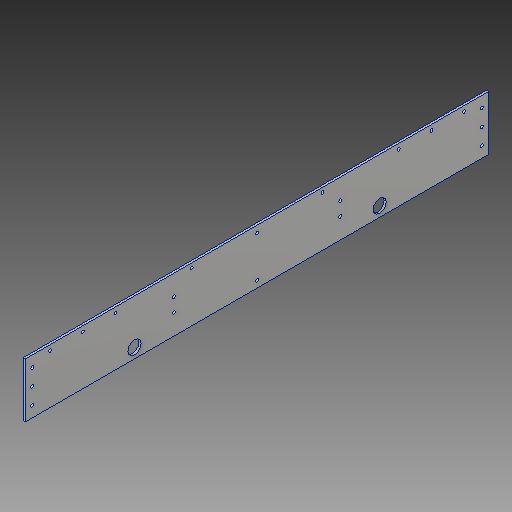
# Autodesk Inventor part: Bumper Plate
Saved by Autodesk Inventor 2019.4 (Build 234330000, 330)
## iProperties
Created: 2019-11-03
Part Number: Bumper Plate
Material: Aluminum 6061
Document SubType Name: Modeling
Designer: admin
Density: 2.7 g/cm^3
Appearance: Aluminum - Flat
Mass: 902.933 g
Surface Area: 1768 cm^2
Volume: 334.42 cm^3
Author: admin
Autodesk Inventor part; units mm, degrees
ref_plane "YZ Plane" through (0, 0, 0) normal (1, 0, 0) x (0, 1, 0)
ref_plane "XZ Plane" through (0, 0, 0) normal (0, 1, 0) x (-1, 0, 0)
ref_plane "XY Plane" through (0, 0, 0) normal (0, 0, 1) x (1, 0, 0)
sketch "Sketch1" plane through (0, 0, 0) normal (1, 0, 0) x (0, 1, 0)
  line L0 (-50, 425) -> (50, 425)
  line L1 (50, 425) -> (50, -425)
  line L2 (50, -425) -> (-50, -425)
  line L3 (-50, -425) -> (-50, 425)
  line L4 (-50, 425) -> (50, -425) construction
  line L5 (50, 425) -> (-50, -425) construction
  point P0 (0, 0)
  dimension "d0" = 100
  dimension "d1" = 850
  constraints: 12 end point, 2 midpoint, 2 parallel, 1 horizontal, 1 perpendicular
  measures "d0" distance of L1.end L2.end
  measures "d1" distance of L0.end L1.end
extrude "Extrusion1" add sketch "Sketch1" along normal blind 4
sketch "Sketch2" plane through (4, 0, 0) normal (1, 0, 0) x (0, 0, -1)
  circle A0 centre (-225, -31.7) radius 12.1
  line L0 (-425, -50) -> (425, -50) projected
  line L1 (-425, 50) -> (-425, -50) projected
  line L2 (425, 50) -> (-425, 50) projected
  line L3 (0, 50) -> (0, -50)
  circle A1 centre (225, -31.7) radius 12.1
  point P0 (0, 0)
  dimension "d4" = 18.3
  dimension "d5" = 200
  dimension "d6" = 24.2
  dimension "d9" = 425
  constraints: 2 centre point, 2 end point, 2 midpoint, 1 perpendicular, 1 symmetric about line, 1 other
  measures "d4" distance from line of L0 A0.centre
  measures "d5" distance from line of L1 A0.centre
  measures "d6" diameter of A0
  measures "d9" distance between parallel lines of L1 L3
extrude "Extrusion2" cut sketch "Sketch2" against normal through all contours A0 | A1
sketch "Sketch3" plane through (4, 0, 0) normal (1, 0, 0) x (0, 0, -1)
  circle A0 centre (120, -42) radius 2.75 projected
  circle A1 centre (120, 42) radius 2.75 projected
  circle A2 centre (0, 37.5) radius 2.75 projected
  circle A3 centre (412.5, 30) radius 2.75 projected
  circle A4 centre (412.5, 0) radius 2.75 projected
  circle A5 centre (412.5, -30) radius 2.75 projected
  circle A6 centre (260, 40.5) radius 2.75 projected
  circle A7 centre (320, 40.5) radius 2.75 projected
  circle A8 centre (145.213, 6.296) radius 10.5 projected
  circle A9 centre (196.913, 6.296) radius 10.5 projected
  circle A10 centre (-145.213, 6.296) radius 10.5 projected
  circle A11 centre (-196.913, 6.296) radius 10.5 projected
  circle A12 centre (-105, -14) radius 10 projected
  circle A13 centre (-79.6, -14) radius 2.75 projected
  circle A14 centre (-130.4, -14) radius 2.75 projected
  circle A15 centre (-264.9997, -22.6996) radius 2.75 projected
  circle A16 centre (-147.163, -33.4172) radius 2.75 projected
  circle A17 centre (264.9997, -22.6996) radius 2.75 projected
  circle A18 centre (174.913, 42.776) radius 2.75 projected
  circle A19 centre (147.163, -33.4172) radius 2.75 projected
  circle A20 centre (130.4, -14) radius 2.75 projected
  circle A21 centre (79.6, -14) radius 2.75 projected
  circle A22 centre (105, 11.4) radius 2.75 projected
  circle A23 centre (105, -39.4) radius 2.75 projected
  circle A24 centre (111.5777, 29.8129) radius 2.75 projected
  circle A25 centre (236.913, 19.219) radius 2.75 projected
  circle A26 centre (-236.913, 19.219) radius 2.75 projected
  circle A27 centre (-174.913, 42.776) radius 2.75 projected
  circle A28 centre (-111.5777, 29.8129) radius 2.75 projected
  circle A29 centre (-105, 11.4) radius 2.75 projected
  circle A30 centre (-105, -39.4) radius 2.75 projected
  circle A31 centre (241, -31.7) radius 2.25 projected
  circle A32 centre (-241, -31.7) radius 2.25 projected
  circle A33 centre (-209, -31.7) radius 2.25 projected
  circle A34 centre (-225, -15.7) radius 2.25 projected
  circle A35 centre (225, -15.7) radius 2.25 projected
  circle A36 centre (209, -31.7) radius 2.25 projected
  circle A37 centre (-225, -31.7) radius 12.3 projected
  circle A38 centre (225, -31.7) radius 12.3 projected
  line L0 (-425, 50) -> (-425, -50) projected
  line L1 (-425, 50) -> (425, 50) projected
  line L2 (425, -50) -> (425, 50) projected
  line L3 (-425, -50) -> (425, -50) projected
  circle A39 centre (-152.5, 12.5) radius 2.75 projected
  circle A40 centre (152.5, 12.5) radius 2.75 projected
  circle A41 centre (152.5, -12.5) radius 2.75 projected
  circle A42 centre (-152.5, -12.5) radius 2.75 projected
  circle A43 centre (0, -37.5) radius 2.75 projected
  circle A44 centre (320, 40.5) radius 2.75 projected
  circle A45 centre (260, 40.5) radius 2.75 projected
  circle A46 centre (0, 37.5) radius 2.75 projected
  circle A47 centre (120, 42) radius 2.75 projected
  circle A48 centre (380, 40.5) radius 2.75 projected
  circle A49 centre (412.5, 0) radius 2.75 projected
  circle A50 centre (412.5, -30) radius 2.75 projected
  circle A51 centre (-264.9997, -22.6996) radius 2.75 projected
  circle A52 centre (-147.163, -33.4172) radius 2.75 projected
  circle A53 centre (264.9997, -22.6996) radius 2.75 projected
  circle A54 centre (174.913, 42.776) radius 2.75 projected
  circle A55 centre (147.163, -33.4172) radius 2.75 projected
  circle A56 centre (111.5777, 29.8129) radius 2.75 projected
  circle A57 centre (236.913, 19.219) radius 2.75 projected
  circle A58 centre (-236.913, 19.219) radius 2.75 projected
  circle A59 centre (-174.913, 42.776) radius 2.75 projected
  circle A60 centre (-111.5777, 29.8129) radius 2.75 projected
  circle A61 centre (225, -31.7) radius 16.3 projected
  circle A62 centre (-225, -31.7) radius 16.3 projected
  line L4 (-425, -50) -> (-425, 50) projected
  line L5 (-425, -50) -> (425, -50) projected
  line L6 (425, 50) -> (425, -50) projected
  line L7 (-425, 50) -> (425, 50) projected
  circle A63 centre (-120, 42) radius 2.75 projected
  circle A64 centre (-105, -14) radius 34 projected
  circle A65 centre (75.0667, -42) radius 2.75 projected
  circle A66 centre (105, -14) radius 34 projected
  circle A67 centre (152.5, -12.5) radius 7.5 projected
  circle A68 centre (-152.5, -12.5) radius 7.5 projected
  circle A69 centre (-85.6, 40) radius 2.75 projected
  circle A70 centre (15.6, 40) radius 2.75 projected
  circle A71 centre (364.4, 40) radius 2.75 projected
  circle A72 centre (364.5, -40) radius 2.75 projected
  circle A73 centre (15.6, -40) radius 2.75 projected
  circle A74 centre (-85.6, -40) radius 2.75 projected
  arc A75 (-119.576, -44.7171) -> (-92.3554, -45.5613) centre (-105, -14) ccw projected
  circle A76 centre (15.6, -40) radius 8.75 projected
  circle A77 centre (-85.6, 40) radius 8.75 projected
  circle A78 centre (15.6, 40) radius 8.75 projected
  circle A79 centre (364.5, -40) radius 8.75 projected
  arc A80 (-92.3554, -45.5613) -> (-78.3455, -35.1077) centre (-85.6, -40) ccw projected
  circle A81 centre (105, -14) radius 10 projected
  circle A82 centre (0, 0) radius 25 projected
  circle A83 centre (0, 0) radius 25 projected
  arc A84 (119.576, -44.7171) -> (122.4969, -43.1523) centre (120, -42) ccw projected
  arc A85 (122.4969, -43.1523) -> (119.576, -44.7171) centre (105, -14) ccw projected
  arc A86 (-78.3455, -35.1077) -> (-122.4969, -43.1523) centre (-105, -14) ccw projected
  circle A87 centre (412.5, 30) radius 2.75 projected
  circle A88 centre (412.5, 30) radius 2.75 projected
  circle A89 centre (364.4, 40) radius 8.75 projected
  circle A90 centre (364.4, 40) radius 8.75 projected
  circle A91 centre (0, -37.5) radius 7.75 projected
  circle A92 centre (380, 40.5) radius 6.75 projected
  circle A93 centre (-412.5, 0) radius 2.75 projected
  circle A94 centre (-380, 40.5) radius 2.75 projected
  circle A95 centre (-260, 40.5) radius 2.75 projected
  circle A96 centre (-320, 40.5) radius 2.75 projected
  circle A97 centre (-412.5, 30) radius 2.75 projected
  circle A98 centre (-412.5, -30) radius 2.75 projected
  circle A99 centre (-120, -42) radius 2.75 projected
  arc A100 (-122.4969, -43.1523) -> (-119.576, -44.7171) centre (-120, -42) ccw projected
  circle A101 centre (-412.5, -30) radius 2.75 projected
  circle A102 centre (-412.5, 30) radius 2.75 projected
  circle A103 centre (-320, 40.5) radius 2.75 projected
  circle A104 centre (-260, 40.5) radius 2.75 projected
  circle A105 centre (-380, 40.5) radius 2.75 projected
  circle A106 centre (-412.5, 0) radius 2.75 projected
  circle A107 centre (-120, 42) radius 2.75 projected
  point P0 (0, 0)
  point P1 (72.4969, -43.1523)
  point P2 (69.576, -44.7171)
  point P3 (369.0669, 32.5985)
  point P4 (365.7758, 31.3588)
  point P5 (368.1667, 30)
  point P6 (-105, -14)
  point P7 (-105, -14)
  point P8 (105, -14)
  point P9 (-105, -14)
  point P10 (-105, -14)
  constraints: 2 other
extrude "Extrusion3" cut sketch "Sketch3" against normal blind 10 contours A1 | A2 | A4 | A5 | A6 | A7 | A40 A8 | A8 A40 | A39 A10 | A10 A39 | A41 | A42 | A43 picked at (152.3295, 12.2121) picked at (153.6603, 13.4669) picked at (-152.2792, 12.2624) picked at (-153.718, 13.3887)
sketch "Sketch4" plane through (4, 0, 0) normal (1, 0, 0) x (0, 0, -1)
  circle A0 centre (120, 42) radius 2.75 projected
  circle A1 centre (0, 37.5) radius 2.75 projected
  circle A2 centre (-120, 42) radius 2.75 projected
  circle A3 centre (152.5, 12.5) radius 2.75 projected
  circle A4 centre (152.5, -12.5) radius 2.75 projected
  circle A5 centre (-152.5, 12.5) radius 2.75 projected
  circle A6 centre (-152.5, -12.5) radius 2.75 projected
  circle A7 centre (-412.5, 30) radius 2.75 projected
  circle A8 centre (-412.5, 0) radius 2.75 projected
  circle A9 centre (-412.5, -30) radius 2.75 projected
  circle A10 centre (412.5, 30) radius 2.75 projected
  circle A11 centre (412.5, 0) radius 2.75 projected
  circle A12 centre (412.5, -30) radius 2.75 projected
  circle A13 centre (380, 40.5) radius 2.75 projected
  circle A14 centre (320, 40.5) radius 2.75 projected
  circle A15 centre (260, 40.5) radius 2.75 projected
  circle A16 centre (-380, 40.5) radius 2.75 projected
  circle A17 centre (-320, 40.5) radius 2.75 projected
  circle A18 centre (-260, 40.5) radius 2.75 projected
  point P0 (0, 0)
extrude "Extrusion4" cut sketch "Sketch4" against normal through all
body "Solid1"
